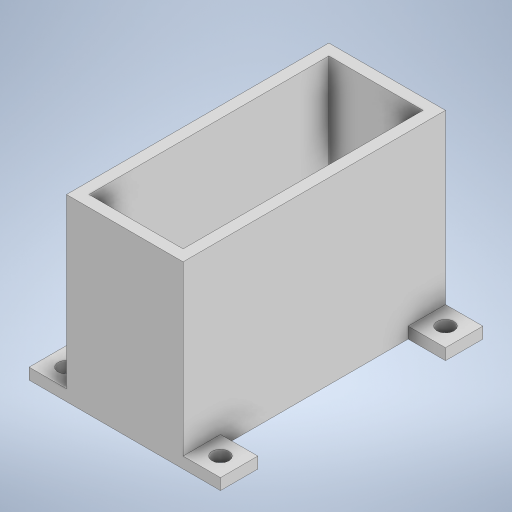
# Autodesk Inventor part: rasp_battery_fastening
Saved by Autodesk Inventor 2024 (Build 280153000, 153)
## iProperties
Created: 2024-05-18
Part Number: rasp_battery_fastening
Material: Generic
Document SubType Name: Modeling
Designer: inigo
Density: 1 g/cm^3
Appearance: Default
Author: inigo
Autodesk Inventor part; units mm, degrees
ref_plane "YZ Plane" through (0, 0, 0) normal (1, 0, 0) x (0, 1, 0)
ref_plane "XZ Plane" through (0, 0, 0) normal (0, 1, 0) x (-1, 0, 0)
ref_plane "XY Plane" through (0, 0, 0) normal (0, 0, 1) x (1, 0, 0)
sketch "Sketch1" plane through (0, 0, 0) normal (0, 1, 0) x (-1, 0, 0)
  line L0 (12.6, 32.1) -> (-12.6, 32.1)
  line L1 (-12.6, 32.1) -> (-12.6, -32.1)
  line L2 (-12.6, -32.1) -> (12.6, -32.1)
  line L3 (12.6, -32.1) -> (12.6, 32.1)
  line L4 (12.6, 32.1) -> (-12.6, -32.1) construction
  line L5 (-12.6, 32.1) -> (12.6, -32.1) construction
  line L6 (15.6, 35.1) -> (-15.6, 35.1)
  line L7 (-15.6, 35.1) -> (-15.6, -35.1)
  line L8 (-15.6, -35.1) -> (15.6, -35.1)
  line L9 (15.6, -35.1) -> (15.6, 35.1)
  point P0 (0, 0)
  dimension "d0" = 25.2
  dimension "d1" = 64.2
  dimension "d2" = 3
  constraints: 20 end point, 4 parallel, 2 midpoint, 2 perpendicular, 1 horizontal, 3 other
  measures "d0" distance of L2.end L1.end
  measures "d1" distance of L1.end L0.end
  measures "d2" distance between parallel lines of L3 L9
extrude "Extrusion1" add sketch "Sketch1" along normal blind 45
sketch "Sketch2" plane through (0, 0, 0) normal (0, -1, 0) x (1, 0, 0)
  circle A0 centre (20.6, 30.1) radius 2.25
  line L0 (-15.6, 35.1) -> (15.6, 35.1) projected
  line L1 (15.6, 35.1) -> (25.6, 35.1)
  line L2 (25.6, 35.1) -> (25.6, 25.1)
  line L3 (25.6, 25.1) -> (15.6, 25.1)
  line L4 (15.6, 25.1) -> (15.6, 35.1)
  line L5 (15.6, 35.1) -> (15.6, -35.1) projected
  line L6 (15.6, 0) -> (48.6737, 0)
  line L7 (15.6, -35.1) -> (-15.6, -35.1) projected
  line L8 (0, -35.1) -> (0, -68.9051)
  circle A1 centre (20.6, -30.1) radius 2.25
  line L9 (15.6, -35.1) -> (25.6, -35.1)
  line L10 (25.6, -35.1) -> (25.6, -25.1)
  line L11 (25.6, -25.1) -> (15.6, -25.1)
  line L12 (15.6, -25.1) -> (15.6, -35.1)
  circle A2 centre (-20.6, 30.1) radius 2.25
  line L13 (-15.6, 35.1) -> (-25.6, 35.1)
  line L14 (-25.6, 35.1) -> (-25.6, 25.1)
  line L15 (-25.6, 25.1) -> (-15.6, 25.1)
  line L16 (-15.6, 25.1) -> (-15.6, 35.1)
  circle A3 centre (-20.6, -30.1) radius 2.25
  line L17 (-15.6, -35.1) -> (-25.6, -35.1)
  line L18 (-25.6, -35.1) -> (-25.6, -25.1)
  line L19 (-25.6, -25.1) -> (-15.6, -25.1)
  line L20 (-15.6, -25.1) -> (-15.6, -35.1)
  line L21 (-15.6, 35.1) -> (15.6, 35.1)
  line L22 (15.6, 35.1) -> (15.6, -35.1)
  line L23 (15.6, -35.1) -> (-15.6, -35.1)
  line L24 (-15.6, -35.1) -> (-15.6, 35.1)
  point P0 (0, 0)
  point P1 (15.6, 30.1)
  point P2 (15.6, -30.1)
  point P3 (-15.6, 30.1)
  point P4 (-15.6, -30.1)
  dimension "d5" = 4.5
  dimension "d6" = 10
  dimension "d7" = 10
  dimension "d8" = 5
  dimension "d9" = 5
  constraints: 44 end point, 15 symmetric about line, 4 centre point, 4 parallel, 3 horizontal, 3 midpoint, 2 perpendicular, 1 vertical, 3 other
  measures "d5" diameter of A0
  measures "d6" distance of L2.end L3.end
  measures "d7" distance of L1.end L2.end
  measures "d8" distance of point (15.6, 30.1) A0.centre
  measures "d9" distance from line of L1 A0.centre
extrude "Extrusion2" add sketch "Sketch2" along normal blind 3
body "Solid1"
